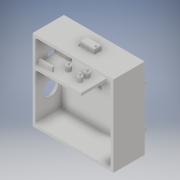
# Autodesk Inventor part: Box
Saved by Autodesk Inventor 2018.2 (Build 222227000, 227)
## iProperties
Created: 2018-04-19
Part Number: Box
Material: Generic
Document SubType Name: Modeling
Designer: MIABo
Density: 1 g/cm^3
Appearance: Default
Author: MIABo
Autodesk Inventor part; units mm, degrees
ref_plane "YZ Plane" through (0, 0, 0) normal (1, 0, 0) x (0, 1, 0)
ref_plane "XZ Plane" through (0, 0, 0) normal (0, 1, 0) x (-1, 0, 0)
ref_plane "XY Plane" through (0, 0, 0) normal (0, 0, 1) x (1, 0, 0)
sketch "Sketch1" plane through (0, 0, 0) normal (0, 0, 1) x (1, 0, 0)
  line L0 (0, 0) -> (-114.3, 0)
  line L1 (-114.3, 0) -> (-114.3, 114.3)
  line L2 (-114.3, 114.3) -> (0, 114.3)
  line L3 (0, 114.3) -> (0, 0)
  dimension "d0" = 114.3
  dimension "d1" = 114.3
  constraints: 8 end point, 2 parallel, 1 horizontal, 1 perpendicular
  measures "d0" distance of L1.end L2.end
  measures "d1" distance of L0.end L1.end
extrude "Extrusion1" add sketch "Sketch1" along normal blind 6.35
sketch "Sketch2" plane through (0, 0, 6.35) normal (0, 0, 1) x (1, 0, 0)
  line L0 (-110.49, 110.49) -> (-3.81, 110.49)
  line L1 (-3.81, 110.49) -> (-3.81, 3.81)
  line L2 (-3.81, 3.81) -> (-110.49, 3.81)
  line L3 (-110.49, 3.81) -> (-110.49, 110.49)
  line L4 (-114.3, 114.3) -> (-114.3, 0) projected
  line L5 (-114.3, 114.3) -> (0, 114.3)
  line L6 (0, 114.3) -> (0, 0)
  line L7 (0, 0) -> (-114.3, 0)
  line L8 (-114.3, 0) -> (-114.3, 114.3)
  dimension "d5" = 3.81
  dimension "d6" = 3.81
  dimension "d7" = 3.81
  dimension "d8" = 3.81
  constraints: 16 end point, 4 parallel, 2 horizontal, 2 perpendicular
  measures "d5" distance between parallel lines of L5 L0
  measures "d6" distance between parallel lines of L6 L1
  measures "d7" distance between parallel lines of L7 L2
  measures "d8" distance between parallel lines of L4 L3
extrude "Extrusion2" add sketch "Sketch2" along normal blind 38.1
sketch "Sketch3" plane through (0, 0, 0) normal (0, 0, -1) x (-1, 0, 0)
  circle A0 centre (109.22, 85.725) radius 3.175
  circle A1 centre (109.22, 28.575) radius 3.175
  line L0 (114.3, 0) -> (114.3, 114.3) projected
  line L1 (114.3, 114.3) -> (0, 114.3) projected
  circle A2 centre (5.08, 85.725) radius 3.175
  circle A3 centre (5.08, 28.575) radius 3.175
  line L2 (0, 114.3) -> (0, 0) projected
  line L3 (0, 0) -> (114.3, 0) projected
  dimension "d11" = 6.35
  dimension "d21" = 57.15
  dimension "d24" = 57.15
  dimension "d25" = 104.14
  dimension "d26" = 104.14
  dimension "d27" = 28.575
  dimension "d29" = 114.3
  dimension "d30" = 5.08
  dimension "d31" = 5.08
  dimension "d32" = 5.08
  constraints: 4 centre point, 3 equal radius
  measures "d11" diameter of A0
  measures "d21" distance of A3.centre A2.centre
  measures "d24" distance of A1.centre A0.centre
  measures "d25" distance of A2.centre A0.centre
  measures "d26" distance of A3.centre A1.centre
  measures "d27" distance from line of L1 A0.centre
  measures "d29" distance of L0.start L0.end
  measures "d30" distance from line of A0.centre L0
  measures "d31" distance from line of L2 A3.centre
  measures "d32" distance from line of L0 A1.centre
extrude "Extrusion3" add sketch "Sketch3" along normal blind 5.08 contours A0 | A1 | A2 | A3
sketch "Sketch4" plane through (0, 0, 0) normal (0, 0, -1) x (-1, 0, 0)
  line L0 (0, 114.3) -> (0, 0) projected
  line L1 (114.3, 114.3) -> (0, 114.3) projected
  point P0 (57.15, 57.15)
  dimension "d35" = 57.15
  dimension "d36" = 57.15
  measures "d35" distance from line of L0 point (57.15, 57.15)
  measures "d36" distance from line of L1 point (57.15, 57.15)
hole "Hole1" at (-57.15, 57.15, 0) direction (0, 0, 1) diameter 6.35 end up to face face through (-74.93, 74.93, 6.35) facing (0, 0, 1)
sketch "Sketch5" plane through (0, 0, 6.35) normal (0, 0, 1) x (1, 0, 0)
  line L0 (-110.49, 110.49) -> (-110.49, 3.81) projected
  line L1 (-110.49, 74.93) -> (-45.72, 74.93)
  line L2 (-45.72, 74.93) -> (-45.72, 71.12)
  line L3 (-45.72, 71.12) -> (-110.49, 71.12)
  line L4 (-110.49, 71.12) -> (-110.49, 74.93)
  line L5 (-110.49, 110.49) -> (-3.81, 110.49) projected
  point P0 (0, 0)
  dimension "d60" = 64.77
  dimension "d61" = 3.81
  dimension "d62" = 106.68
  dimension "d63" = 35.56
  constraints: 8 end point, 2 parallel, 1 horizontal, 1 perpendicular, 1 point on line
  measures "d60" distance of L2.end L3.end
  measures "d61" distance of L1.end L2.end
  measures "d62" distance of L0.start L0.end
  measures "d63" distance between parallel lines of L5 L1
sketch "Sketch6" plane through (-114.3, 114.3, 0) normal (0, 1, 0) x (1, 0, 0)
  line L0 (47.498, -17.145) -> (70.358, -17.145)
  line L1 (70.358, -17.145) -> (70.358, -27.305)
  line L2 (70.358, -27.305) -> (47.498, -27.305)
  line L3 (47.498, -27.305) -> (47.498, -17.145)
  circle A0 centre (67.818, -22.225) radius 1.524
  line L4 (0, 0) -> (0, -44.45) projected
  line L5 (114.3, -44.45) -> (0, -44.45) projected
  point P0 (114.3, 0)
  point P1 (57.15, -22.225)
  dimension "d44" = 22.86
  dimension "d45" = 10.16
  dimension "d46" = 3.048
  dimension "d47" = 5.08
  dimension "d48" = 2.54
  dimension "d49" = 5.08
  dimension "d50" = 9.652
  dimension "d51" = 57.15
  dimension "d52" = 44.45
  dimension "d53" = 22.225
  constraints: 8 end point, 2 parallel, 1 centre point, 1 horizontal, 1 perpendicular
  measures "d44" distance of L1.end L2.end
  measures "d45" distance of L0.end L1.end
  measures "d46" diameter of A0
  measures "d47" distance from line of L2 A0.centre
  measures "d48" distance from line of L1 A0.centre
  measures "d49" distance from line of L2 point (57.15, -22.225)
  measures "d50" distance from line of L3 point (57.15, -22.225)
  measures "d51" distance from line of L4 point (57.15, -22.225)
  measures "d52" distance of L4.start L4.end
  measures "d53" distance from line of L5 point (57.15, -22.225)
extrude "Extrusion4" add sketch "Sketch6" along normal blind 6.35
sketch "Sketch7" plane through (-114.3, 120.65, 0) normal (0, 1, 0) x (1, 0, 0)
  line L0 (47.498, -17.145) -> (47.498, -27.305) projected
  line L1 (70.358, -27.305) -> (47.498, -27.305) projected
  line L2 (47.498, -17.145) -> (50.038, -17.145)
  line L3 (50.038, -17.145) -> (50.038, -27.305)
  line L4 (50.038, -27.305) -> (47.498, -27.305)
  line L5 (47.498, -27.305) -> (47.498, -17.145)
  point P0 (114.3, 0)
  dimension "d56" = 2.54
  constraints: 8 end point, 2 parallel, 1 horizontal, 1 perpendicular, 1 point on line
  measures "d56" distance of L3.end L4.end
extrude "Extrusion5" cut sketch "Sketch7" against normal up to surface (10.16 mm away)
fillet "Fillet1" radius 3.175 4 edges at (-110.49, 110.49, 25.4) (-3.81, 110.49, 25.4) (-110.49, 3.81, 25.4) (-3.81, 3.81, 25.4)
extrude "Extrusion6" add sketch "Sketch5" along normal up to surface (38.1 mm away)
sketch "Sketch8" plane through (-110.49, 74.93, 6.35) normal (0, 1, 0) x (1, 0, 0)
  circle A0 centre (27.94, -19.05) radius 1.524
  circle A1 centre (49.2125, -24.13) radius 1.524
  circle A2 centre (49.2125, -13.97) radius 1.524
  line L0 (0, -38.1) -> (64.77, -38.1) projected
  point P0 (110.49, 6.35)
  dimension "d66" = 3.048
  dimension "d67" = 27.94
  dimension "d68" = 10.16
  dimension "d69" = 19.05
  dimension "d70" = 13.97
  constraints: 3 centre point, 2 equal radius
  measures "d66" diameter of A0
  measures "d67" horizontal distance of A0.centre L0.start
  measures "d68" distance of A1.centre A2.centre
  measures "d69" distance from line of L0 A0.centre
  measures "d70" distance from line of L0 A1.centre
extrude "Extrusion7" add sketch "Sketch8" along normal blind 10.16
sketch "Sketch9" plane through (-110.49, 74.93, 6.35) normal (0, 1, 0) x (1, 0, 0)
  circle A0 centre (27.94, -19.05) radius 1.524 projected
  circle A1 centre (27.94, -19.05) radius 3.4925
  circle A2 centre (49.2125, -24.13) radius 1.524 projected
  circle A3 centre (49.2125, -24.13) radius 3.4925
  circle A4 centre (49.2125, -13.97) radius 1.524 projected
  circle A5 centre (49.2125, -13.97) radius 3.4925
  line L0 (0, -33.02) -> (19.05, -33.02)
  line L1 (19.05, -33.02) -> (19.05, -30.48)
  line L2 (19.05, -30.48) -> (0, -30.48)
  line L3 (0, -30.48) -> (0, -33.02)
  line L4 (0, -5.08) -> (19.05, -5.08)
  line L5 (19.05, -5.08) -> (19.05, -7.62)
  line L6 (19.05, -7.62) -> (0, -7.62)
  line L7 (0, -7.62) -> (0, -5.08)
  line L8 (0, -38.1) -> (0, 0) projected
  point P0 (110.49, 6.35)
  dimension "d73" = 6.985
  dimension "d74" = 27.94
  dimension "d75" = 13.97
  dimension "d76" = 19.05
  dimension "d77" = 2.54
  dimension "d78" = 2.54
  constraints: 16 end point, 4 parallel, 3 centre point, 3 coincident, 2 equal radius, 2 horizontal, 2 perpendicular, 2 point on line, 1 collinear
  measures "d73" diameter of A1
  measures "d74" distance between parallel lines of L0 L4
  measures "d75" distance from line of L0 A1.centre
  measures "d76" distance of L0.start L0.end
  measures "d77" distance of L1.end L0.end
  measures "d78" distance of L6.end L4.start
extrude "Extrusion8" add sketch "Sketch9" along normal blind 6.35
fillet "Fillet2" radius 3.175 7 edges at (-78.105, 74.93, 6.35) (-78.105, 71.12, 6.35) (-110.49, 71.12, 25.4) (-110.49, 74.93, 25.4) (-110.49, 74.93, 41.91) (-110.49, 74.93, 8.89) (-45.72, 73.025, 6.35)
sketch "Sketch10" plane through (-110.49, 107.315, 44.45) normal (1, 0, 0) x (0, 0, -1)
  line L0 (30.48, -23.495) -> (17.78, -23.495)
  line L1 (17.78, -23.495) -> (17.78, -32.385)
  line L2 (17.78, -32.385) -> (30.48, -32.385)
  line L3 (30.48, -32.385) -> (30.48, -23.495)
  line L4 (7.62, -32.385) -> (30.48, -32.385) projected
  point P0 (44.45, -107.315)
  point P1 (33.02, -26.035)
  point P2 (5.08, -26.035)
  point P3 (24.13, -26.035)
  dimension "d82" = 12.7
  dimension "d83" = 8.89
  dimension "d84" = 2.54
  dimension "d85" = 27.94
  dimension "d86" = 8.89
  constraints: 8 end point, 2 parallel, 1 collinear, 1 horizontal, 1 perpendicular
  measures "d82" distance of L0.start L0.end
  measures "d83" distance of L0.end L1.end
  measures "d84" distance from line of L3 point (33.02, -26.035)
  measures "d85" distance of point (33.02, -26.035) point (5.08, -26.035)
  measures "d86" distance of point (24.13, -26.035) point (33.02, -26.035)
extrude "Extrusion9" cut sketch "Sketch10" against normal blind 6.35 and the other way blind 3.175
sketch "Sketch11" plane through (-114.3, 0, 0) normal (-1, 0, 0) x (0, 0, 1)
  line L0 (44.45, 114.3) -> (44.45, 0) projected
  line L1 (0, 0) -> (0, 114.3) projected
  line L2 (13.97, 83.82) -> (26.67, 83.82) projected
  line L3 (12.573, 92.3951) -> (28.067, 92.3951) construction
  line L4 (28.067, 92.3951) -> (28.067, 84.3312) construction
  line L5 (28.067, 84.3312) -> (12.573, 84.3312) construction
  line L6 (12.573, 84.3312) -> (12.573, 92.3951) construction
  line L7 (13.97, 74.93) -> (13.97, 83.82) projected
  spline S0 degree 2 poles (15.4341, 85.7981) (14.8732, 85.7981) (14.0396, 86.0914) (13.7463, 86.3847) knots 0 0 0 1 2 2 2
  spline S1 degree 2 poles (13.7463, 86.3847) (13.4118, 86.7141) (13.139, 87.6403) (13.139, 88.3196) knots 0 0 0 1 2 2 2
  line L8 (13.139, 88.3196) -> (13.139, 92.2819)
  line L9 (13.139, 92.2819) -> (13.983, 92.2819)
  line L10 (13.983, 92.2819) -> (13.983, 88.3196)
  spline S2 degree 2 poles (13.983, 88.3196) (13.983, 87.877) (14.0962, 87.2801) (14.2557, 87.0383) knots 0 0 0 1 2 2 2
  spline S3 degree 2 poles (14.2557, 87.0383) (14.4255, 86.781) (15.0121, 86.5185) (15.4341, 86.5185) knots 0 0 0 1 2 2 2
  spline S4 degree 2 poles (15.4341, 86.5185) (15.8303, 86.5185) (16.4478, 86.781) (16.6177, 87.0383) knots 0 0 0 1 2 2 2
  spline S5 degree 2 poles (16.6177, 87.0383) (16.7772, 87.2801) (16.8904, 87.8719) (16.8904, 88.299) knots 0 0 0 1 2 2 2
  line L11 (16.8904, 88.299) -> (16.8904, 92.2819)
  line L12 (16.8904, 92.2819) -> (17.7343, 92.2819)
  line L13 (17.7343, 92.2819) -> (17.7343, 88.3196)
  spline S6 degree 2 poles (17.7343, 88.3196) (17.7343, 87.6558) (17.4667, 86.7089) (17.1271, 86.3847) knots 0 0 0 1 2 2 2
  spline S7 degree 2 poles (17.1271, 86.3847) (16.8235, 86.0863) (16.0207, 85.7981) (15.4341, 85.7981) knots 0 0 0 1 2 2 2
  spline S8 degree 2 poles (20.7138, 85.8187) (20.0242, 85.8187) (19.0568, 86.1069) (18.6297, 86.3127) knots 0 0 0 1 2 2 2
  line L14 (18.6297, 86.3127) -> (18.6297, 87.3727)
  line L15 (18.6297, 87.3727) -> (18.6914, 87.3727)
  spline S9 degree 2 poles (18.6914, 87.3727) (19.1083, 86.9817) (20.1632, 86.5494) (20.652, 86.5494) knots 0 0 0 1 2 2 2
  spline S10 degree 2 poles (20.652, 86.5494) (21.3518, 86.5494) (22.0671, 87.1309) (22.0671, 87.6095) knots 0 0 0 1 2 2 2
  spline S11 degree 2 poles (22.0671, 87.6095) (22.0671, 87.9902) (21.6915, 88.4637) (21.285, 88.582) knots 0 0 0 1 2 2 2
  spline S12 degree 2 poles (21.285, 88.582) (20.9916, 88.6644) (20.5028, 88.7776) (20.1374, 88.8702) knots 0 0 0 1 2 2 2
  spline S13 degree 2 poles (20.1374, 88.8702) (19.8081, 88.9577) (19.2884, 89.2201) (19.0877, 89.4311) knots 0 0 0 1 2 2 2
  spline S14 degree 2 poles (19.0877, 89.4311) (18.8921, 89.6421) (18.676, 90.2081) (18.676, 90.5786) knots 0 0 0 1 2 2 2
  spline S15 degree 2 poles (18.676, 90.5786) (18.676, 91.3505) (19.8801, 92.3951) (20.8115, 92.3951) knots 0 0 0 1 2 2 2
  spline S16 degree 2 poles (20.8115, 92.3951) (21.3467, 92.3951) (22.2935, 92.1841) (22.7001, 91.9834) knots 0 0 0 1 2 2 2
  line L16 (22.7001, 91.9834) -> (22.7001, 90.9748)
  line L17 (22.7001, 90.9748) -> (22.6383, 90.9748)
  spline S17 degree 2 poles (22.6383, 90.9748) (22.3347, 91.2527) (21.3879, 91.6644) (20.8681, 91.6644) knots 0 0 0 1 2 2 2
  spline S18 degree 2 poles (20.8681, 91.6644) (20.2815, 91.6644) (19.5559, 91.1138) (19.5559, 90.6661) knots 0 0 0 1 2 2 2
  spline S19 degree 2 poles (19.5559, 90.6661) (19.5559, 90.2647) (19.983, 89.7862) (20.3844, 89.6781) knots 0 0 0 1 2 2 2
  spline S20 degree 2 poles (20.3844, 89.6781) (20.652, 89.606) (21.429, 89.4208) (21.6863, 89.3436) knots 0 0 0 1 2 2 2
  spline S21 degree 2 poles (21.6863, 89.3436) (22.3399, 89.1429) (22.9471, 88.335) (22.9471, 87.7432) knots 0 0 0 1 2 2 2
  spline S22 degree 2 poles (22.9471, 87.7432) (22.9471, 87.3676) (22.6435, 86.6472) (22.3707, 86.395) knots 0 0 0 1 2 2 2
  spline S23 degree 2 poles (22.3707, 86.395) (22.0671, 86.1171) (21.2952, 85.8187) (20.7138, 85.8187) knots 0 0 0 1 2 2 2
  spline S24 degree 2 poles (28.1135, 87.8822) (28.1135, 87.4088) (27.7533, 86.6832) (27.4548, 86.4465) knots 0 0 0 1 2 2 2
  spline S25 degree 2 poles (27.4548, 86.4465) (27.0946, 86.1686) (26.2764, 85.9319) (25.6281, 85.9319) knots 0 0 0 1 2 2 2
  line L18 (25.6281, 85.9319) -> (23.8064, 85.9319)
  line L19 (23.8064, 85.9319) -> (23.8064, 92.2819)
  line L20 (23.8064, 92.2819) -> (25.4891, 92.2819)
  spline S26 degree 2 poles (25.4891, 92.2819) (26.1684, 92.2819) (26.8476, 92.1944) (27.1564, 92.0246) knots 0 0 0 1 2 2 2
  spline S27 degree 2 poles (27.1564, 92.0246) (27.5012, 91.8445) (27.8151, 91.2527) (27.8151, 90.8513) knots 0 0 0 1 2 2 2
  spline S28 degree 2 poles (27.8151, 90.8513) (27.8151, 90.4037) (27.3416, 89.6935) (26.9248, 89.4928) knots 0 0 0 1 2 2 2
  line L21 (26.9248, 89.4928) -> (26.9248, 89.462)
  spline S29 degree 2 poles (26.9248, 89.462) (27.4909, 89.3076) (28.1135, 88.4894) (28.1135, 87.8822) knots 0 0 0 1 2 2 2
  spline S30 degree 2 poles (27.2336, 87.8462) (27.2336, 88.2064) (27.0277, 88.6695) (26.719, 88.8342) knots 0 0 0 1 2 2 2
  spline S31 degree 2 poles (26.719, 88.8342) (26.5183, 88.9371) (26.0449, 88.9988) (25.6075, 88.9988) knots 0 0 0 1 2 2 2
  line L22 (25.6075, 88.9988) -> (24.6503, 88.9988)
  line L23 (24.6503, 88.9988) -> (24.6503, 86.6523)
  line L24 (24.6503, 86.6523) -> (25.3348, 86.6523)
  spline S32 degree 2 poles (25.3348, 86.6523) (25.8905, 86.6523) (26.5286, 86.7552) (26.7756, 86.9199) knots 0 0 0 1 2 2 2
  spline S33 degree 2 poles (26.7756, 86.9199) (27.0123, 87.0897) (27.2336, 87.5117) (27.2336, 87.8462) knots 0 0 0 1 2 2 2
  spline S34 degree 2 poles (26.9351, 90.733) (26.9351, 90.9594) (26.7807, 91.299) (26.6109, 91.3968) knots 0 0 0 1 2 2 2
  spline S35 degree 2 poles (26.6109, 91.3968) (26.4051, 91.51) (25.9059, 91.5615) (25.4583, 91.5615) knots 0 0 0 1 2 2 2
  line L25 (25.4583, 91.5615) -> (24.6503, 91.5615)
  line L26 (24.6503, 91.5615) -> (24.6503, 89.7038)
  line L27 (24.6503, 89.7038) -> (25.6075, 89.7038)
  spline S36 degree 2 poles (25.6075, 89.7038) (26.0037, 89.7038) (26.3794, 89.7862) (26.5801, 89.9148) knots 0 0 0 1 2 2 2
  spline S37 degree 2 poles (26.5801, 89.9148) (26.7756, 90.0383) (26.9351, 90.4345) (26.9351, 90.733) knots 0 0 0 1 2 2 2
  dimension "d94" = 15.494
  dimension "d95" = 12.7
  dimension "d97" = 1.397
  constraints: 2 other
  measures "d94" distance of L3.start L3.end
  measures "d95" distance of L2.start L2.end
  measures "d97" distance between parallel lines of L6 L7
extrude "Extrusion10" add sketch "Sketch11" along normal blind 1.27
sketch "Sketch12" plane through (-114.3, 0, 0) normal (-1, 0, 0) x (0, 0, 1)
  circle A0 centre (22.225, 38.1) radius 10.16
  line L0 (44.45, 114.3) -> (44.45, 0) projected
  line L1 (0, 0) -> (0, 114.3) projected
  line L2 (0, 0) -> (44.45, 0) projected
  dimension "d100" = 20.32
  dimension "d101" = 44.45
  dimension "d102" = 22.225
  dimension "d103" = 114.3
  dimension "d104" = 38.1
  constraints: 1 centre point
  measures "d100" diameter of A0
  measures "d101" distance between parallel lines of L0 L1
  measures "d102" distance from line of L1 A0.centre
  measures "d103" distance of L0.start L0.end
  measures "d104" distance from line of L2 A0.centre
extrude "Extrusion11" cut sketch "Sketch12" against normal up to surface (3.81 mm away)
equation "\"d6\" = d5"
equation "\"d7\" = d5"
equation "\"d8\" = d5"
equation "\"d21\" = d24"
equation "\"d26\" = d25"
equation "\"d31\" = d30"
equation "\"d32\" = d30"
equation "\"d63\" = 0.333333 * d62"
equation "\"d53\" = 0.5 * d52"
equation "\"d75\" = 0.5 * d74"
equation "\"d78\" = d77"
equation "\"d97\" = -0.5 * d95 + 0.5 * d94"
equation "\"d102\" = 0.5 * d101"
equation "\"d104\" = 0.333333 * d103"
body "Solid1"
